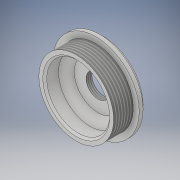
# Autodesk Inventor part: reservoir_cullasse
Saved by Autodesk Inventor 2019 (Build 230136000, 136)
## iProperties
Created: 2019-03-19
Part Number: reservoir_cullasse
Material: Générique
Document SubType Name: Modeling
Designer: theor
Density: 1 g/cm^3
Appearance: Par défaut
Author: theor
Autodesk Inventor part; units mm, degrees
ref_plane "YZ Plane" through (0, 0, 0) normal (1, 0, 0) x (0, 1, 0)
ref_plane "XZ Plane" through (0, 0, 0) normal (0, 1, 0) x (-1, 0, 0)
ref_plane "XY Plane" through (0, 0, 0) normal (0, 0, 1) x (1, 0, 0)
sketch "Esquisse1" plane through (0, 0, 0) normal (1, 0, 0) x (0, 1, 0)
  line L0 (22, 4) -> (22, 0)
  line L1 (22, 4) -> (19, 4)
  line L2 (19, 4) -> (19, 14)
  line L3 (19, 14) -> (16, 14)
  line L4 (16, 14) -> (16, 3)
  line L5 (22, 0) -> (6, 0)
  line L6 (6, 0) -> (6, 3)
  line L7 (6, 3) -> (16, 3)
  line L8 (0, 0) -> (0, -5.3906)
  dimension "d0" = 4
  dimension "d2" = 10
  dimension "d3" = 3
  dimension "d4" = 12
  dimension "d7" = 38
  dimension "d8" = 3
  dimension "d9" = 3
  constraints: 18 end point, 5 vertical, 4 horizontal, 1 horizontal alignment
  measures "d0" distance of L0.end L0.start
  measures "d2" distance of L1.end L2.end
  measures "d3" distance of L5.end L6.end
  measures "d4" diameter of L6 L8
  measures "d7" diameter of L2 L8
  measures "d8" distance between parallel lines of L2 L4
  measures "d9" distance of L0.start L1.end
revolve "Révolution1" add sketch "Esquisse1" angle 360 about axis through (0, 0, 0) along (0, 0, -1)
chamfer "Chanfrein1" distance 2 angle 45 1 edges at (0, -22, 0)
chamfer "Chanfrein2" distance 4 angle 45 1 edges at (0, -16, 3)
thread "Filetage1" size "M38x1.5" class "6g" standard "ISO Metric profile" length 10
chamfer "Chanfrein3" distance 1 angle 45 1 edges at (0, -16, 14)
thread "Filetage2" size "M12x1" class "6H" standard "ISO Metric profile" full length
